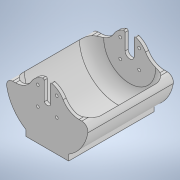
# Autodesk Inventor part: encoder_mount
Saved by Autodesk Inventor 2022.6 (Build 266554010, 554A)
## iProperties
Created: 2025-03-25
Part Number: encoder_mount
Material: 一般
Document SubType Name: Modeling
Designer: gakut
Density: 1 g/cm^3
Appearance: 既定
Author: gakut
## iProperties of the stored document encoder_mount_3D プリント.ipt
Created: 2025-03-25
Part Number: encoder_mount_3D プリント
Material: 一般
Document SubType Name: Modeling
Designer: gakut
Density: 1 g/cm^3
Appearance: 既定
Author: gakut
Autodesk Inventor part; units mm, degrees
ref_plane "YZ Plane" through (0, 0, 0) normal (1, 0, 0) x (0, 1, 0)
ref_plane "XZ Plane" through (0, 0, 0) normal (0, 1, 0) x (-1, 0, 0)
ref_plane "XY Plane" through (0, 0, 0) normal (0, 0, 1) x (1, 0, 0)
sketch "スケッチ1" plane through (0, 0, 0) normal (0, 0, 1) x (1, 0, 0)
  circle A0 centre (0, 0) radius 6
  circle A1 centre (0, 0) radius 67.5
  line L0 (-5, -15) -> (5, -15)
  line L1 (5, -15) -> (5, 15)
  line L2 (5, 15) -> (-5, 15)
  line L3 (-5, 15) -> (-5, -15)
  line L4 (-5, -15) -> (5, 15) construction
  line L5 (5, -15) -> (-5, 15) construction
  point P0 (5, -3.3166)
  point P1 (-5, -3.3166)
  point P2 (-5, 3.3166)
  point P3 (5, 3.3166)
  dimension "d0" = 12
  dimension "d1" = 135
  dimension "d2" = 10
  dimension "d3" = 30
  constraints: 12 end point, 2 centre point, 2 coincident, 2 midpoint, 2 parallel, 1 horizontal, 1 perpendicular
  measures "d0" diameter of A0
  measures "d1" diameter of A1
  measures "d2" distance of L1.end L2.end
  measures "d3" distance of L0.end L1.end
extrude "押し出し1" add sketch "スケッチ1" along normal blind 5 contours A0 L1 | A0 L3 L2 L1 | L1 L0 L3 A0 | L3 A0 | A1
sketch "スケッチ2" plane through (0, 0, 0) normal (0, 0, -1) x (-1, 0, 0)
  arc A0 (5, 3.3166) -> (-5, 3.3166) centre (0, 0) ccw projected
  circle A1 centre (0, 0) radius 62.5
  circle A2 centre (0, 0) radius 67.5
  circle A3 centre (0, 0) radius 67.5 projected
  dimension "d6" = 125
  constraints: 2 centre point, 2 coincident, 1 concentric
  measures "d6" diameter of A1
extrude "押し出し3" add sketch "スケッチ2" along normal blind 130
sketch "スケッチ3" plane through (0, 0, 5) normal (0, 0, 1) x (1, 0, 0)
  circle A0 centre (0, 0) radius 30
  circle A1 centre (0, 0) radius 67.5 projected
  line L0 (-67.5, 0) -> (67.5, 0)
  point P0 (-30, 0)
  point P1 (30, 0)
  dimension "d11" = 60
  constraints: 2 end point, 2 point on circle, 1 centre point, 1 coincident, 1 horizontal, 1 horizontal alignment
  measures "d11" diameter of A0
extrude "押し出し4" cut sketch "スケッチ3" against normal through all contours L0 A0 | L0 A1 A0 | A0 L0 keep common part picked at (1.2054, -54.7734)
sketch "スケッチ4" plane through (0, 0, -130) normal (0, 0, -1) x (-1, 0, 0)
  line L0 (67.5, 0) -> (30, 0) projected
  circle A0 centre (0, 0) radius 67.5
  arc A1 (5, 3.3166) -> (-5, 3.3166) centre (0, 0) ccw projected
  circle A2 centre (0, 0) radius 30
  circle A3 centre (0, 0) radius 7.5
  line L1 (7.5, 0) -> (-7.5, 0)
  line L2 (-7.5, 0) -> (-7.5, 100)
  line L3 (-7.5, 100) -> (7.5, 100)
  line L4 (7.5, 100) -> (7.5, 0)
  line L5 (-30, 0) -> (-67.5, 0) projected
  line L6 (-67.5, 0) -> (67.5, 0)
  point P0 (30, 0)
  point P1 (7.5, 29.0474)
  point P2 (-7.5, 0)
  point P3 (-7.5, 29.0474)
  dimension "d14" = 60
  dimension "d16" = 15
  dimension "d17" = 15
  dimension "d18" = 100
  constraints: 10 end point, 3 coincident, 2 parallel, 1 centre point, 1 collinear, 1 horizontal, 1 horizontal alignment, 1 perpendicular, 1 point on circle, 5 other
  measures "d17" distance of L2.end L3.end
  measures "d18" distance of L1.end L2.end
extrude "押し出し5" add sketch "スケッチ4" along normal blind 5 contours A0 L5 A2 L0 | L6 L4 A2 | A2 L6 A3 | A2 L2 L6
sketch "スケッチ5" plane through (0, 0, -135) normal (0, 0, -1) x (-1, 0, 0)
  line L0 (15.5, 15.5) -> (-15.5, 15.5)
  line L1 (-15.5, 15.5) -> (-15.5, -15.5)
  line L2 (-15.5, -15.5) -> (15.5, -15.5)
  line L3 (15.5, -15.5) -> (15.5, 15.5)
  arc A0 (-5, -3.3166) -> (5, -3.3166) centre (0, 0) ccw projected
  line L4 (15.5, 15.5) -> (-15.5, -15.5) construction
  line L5 (-15.5, 15.5) -> (15.5, -15.5) construction
  dimension "d21" = 31
  dimension "d22" = 31
  constraints: 12 end point, 4 coincident, 2 midpoint, 2 parallel, 1 horizontal, 1 perpendicular
  measures "d21" distance of L2.end L1.end
  measures "d22" distance of L1.end L0.end
hole "穴1" at (-15.5, 15.5, -135) at (15.5, -15.5, -135) at (-15.5, -15.5, -135) at (15.5, 15.5, -135) direction (0, 0, 1) diameter 4.6 end through all
fillet "フィレット1" radius 2 2 edges at (-7.5, 29.0474, -132.5) (7.5, 29.0474, -132.5)
fillet "フィレット2" radius 30 4 edges at (-30, 0, -132.5) (30, 0, -132.5) (30, 0, 2.5) (-30, 0, 2.5)
fillet "フィレット3" radius 10 6 edges at (67.5, 0, -132.5) (67.5, 0, -65) (67.5, 0, 2.5) (-67.5, 0, -132.5) (-67.5, 0, -65) (-67.5, 0, 2.5)
fillet "フィレット4" radius 20 2 edges at (0, -62.5, -130) (0, -62.5, 0)
sketch "スケッチ6" plane through (0, 0, -135) normal (0, 0, -1) x (-1, 0, 0)
  line L0 (-35, -67.5) -> (35, -67.5)
  arc A0 (-66.4714, -11.7391) -> (66.4714, -11.7391) centre (0, 0) ccw projected
  line L1 (-35, -67.5) -> (35, -67.5)
  line L2 (35, -67.5) -> (35, -52.5)
  line L3 (35, -52.5) -> (-35, -52.5)
  line L4 (-35, -52.5) -> (-35, -67.5)
  point P0 (-35, -57.717)
  point P1 (0, -67.5)
  point P2 (35, -57.717)
  dimension "d34" = 70
  dimension "d35" = 35
  dimension "d36" = 15
  constraints: 10 end point, 2 horizontal, 2 parallel, 1 perpendicular, 1 tangent, 1 vertical alignment
  measures "d34" distance of L0.start L0.end
  measures "d35" horizontal distance of point (0, 0) L0.start
  measures "d36" distance of L1.end L2.end
extrude "押し出し6" add sketch "スケッチ6" against normal up to surface (140 mm away) contours L4 A0 L0 | A0 L2 L0
sketch "スケッチ7" plane through (0, 0, 5) normal (0, 0, 1) x (1, 0, 0)
  arc A0 (-5, -3.3166) -> (5, -3.3166) centre (0, 0) ccw projected
  line L0 (-5, -3.3166) -> (5, -3.3166)
  line L1 (5, -3.3166) -> (5, 46.6834)
  line L2 (5, 46.6834) -> (-5, 46.6834)
  line L3 (-5, 46.6834) -> (-5, -3.3166)
  point P0 (5, 3.3166)
  dimension "d39" = 50
  constraints: 8 end point, 2 parallel, 1 horizontal, 1 perpendicular, 1 vertical alignment
  measures "d39" distance of L0.end L1.end
extrude "押し出し7" cut sketch "スケッチ7" against normal blind 10 contours L3 L2 L1 L0
fillet "フィレット5" radius 2 2 edges at (-5, 29.5804, 2.5) (5, 29.5804, 2.5)
equation "\"d17\" = d16"
equation "\"d35\" = 0.5 * d34"
